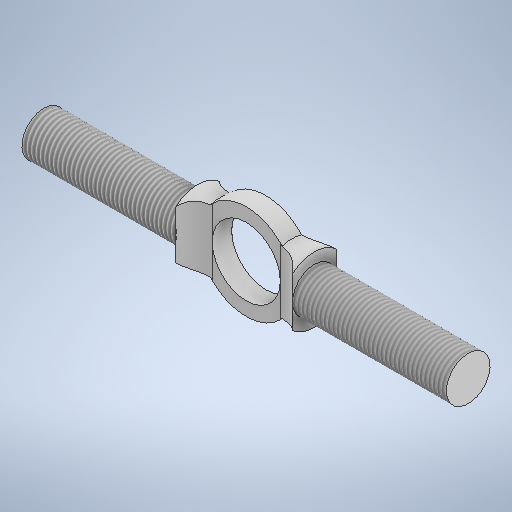
# Autodesk Inventor part: Schraubbolzen
Saved by Autodesk Inventor 2025.2 (Build 292293000, 293)
## iProperties
Created: 2025-02-03
Part Number: Schraubbolzen
Material: Generisch
Document SubType Name: Modeling
Designer: unter
Density: 1 g/cm^3
Appearance: Vorgabe
Author: unter
Autodesk Inventor part; units mm, degrees
ref_plane "YZ Plane" through (0, 0, 0) normal (1, 0, 0) x (0, 1, 0)
ref_plane "XZ Plane" through (0, 0, 0) normal (0, 1, 0) x (-1, 0, 0)
ref_plane "XY Plane" through (0, 0, 0) normal (0, 0, 1) x (1, 0, 0)
derived "Skelett_Laufkatze.ipt"
sketch "Schraubbolzen_oben" plane through (0, 0, -80) normal (0, 0, -1) x (-1, 0, 0)
  line L0 (181, -33.75) -> (131, -33.75) construction
  line L1 (131, -22.5) -> (181, -22.5) construction
  line L2 (131, 22.5) -> (181, 22.5) construction
  line L3 (131, 33.75) -> (181, 33.75) construction
  line L4 (-166, -33.75) -> (-116, -33.75) construction
  line L5 (-116, -22.5) -> (-166, -22.5) construction
  line L6 (-116, 22.5) -> (-166, 22.5) construction
  line L7 (-116, 33.75) -> (-166, 33.75) construction
  line L8 (218.5, 0) -> (-218.5, 0)
  circle A0 centre (0, 0) radius 35
  line L9 (218.5, 0) -> (218.5, 22.5)
  line L10 (218.5, 22.5) -> (60, 22.5)
  line L11 (60, 22.5) -> (60, 33.75)
  line L12 (60, 33.75) -> (36.8909, 33.75)
  line L13 (-36.8909, 33.75) -> (-60, 33.75)
  line L14 (-60, 33.75) -> (-60, 22.5)
  line L15 (-60, 22.5) -> (-218.5, 22.5)
  line L16 (-218.5, 22.5) -> (-218.5, 0)
  line L17 (0, 0) -> (0, 50) construction
  arc A1 (50, 0) -> (-50, 0) centre (0, 0) ccw
  point P0 (-35, 0)
  point P1 (35, 0)
sketch "Schraubbolzen_Ankerausschnitt" plane through (0, 0, -80) normal (0, 1, 0) x (-1, 0, 0)
  line L0 (218.5, 0) -> (-218.5, 0) construction
  line L1 (-35, 0) -> (35, 0) construction
  line L2 (60, 0) -> (36.8909, 0) construction
  line L3 (35, 10) -> (-35, 10)
  line L4 (-35, 10) -> (-35, -10)
  line L5 (-35, -10) -> (35, -10)
  line L6 (35, -10) -> (35, 10)
  line L7 (0, 10) -> (0, -10) construction
  arc A0 (35, 10) -> (60, 22.5) centre (35, 41.25) ccw
  arc A1 (60, -22.5) -> (35, -10) centre (35, -41.25) ccw
  arc A2 (-60, 22.5) -> (-35, 10) centre (-35, 41.25) ccw
  arc A3 (-35, -10) -> (-60, -22.5) centre (-35, -41.25) ccw
  line L8 (60, 22.5) -> (60, 41.25)
  line L9 (60, 41.25) -> (-60, 41.25)
  line L10 (-60, 41.25) -> (-60, 22.5)
  line L11 (60, -22.5) -> (60, -41.25)
  line L12 (60, -41.25) -> (-60, -41.25)
  line L13 (-60, -41.25) -> (-60, -22.5)
  point P0 (0, 80)
  point P1 (-60, 0)
  point P2 (0, 0)
revolve "Umdrehung1" add sketch "Schraubbolzen_oben" angle 360 about axis through (-218.5, 0, -80) along (1, 0, 0) contours L8 A1 L12 L11 L10 L9 | L8 A0 A1 | A1 L8 L16 L15 L14 L13
extrude "Extrusion1" cut sketch "Schraubbolzen_oben" along normal through all both and the other way through all contours A0 L8 | L8 A0
extrude "Extrusion2" cut sketch "Schraubbolzen_Ankerausschnitt" along normal through all both and the other way through all contours L3 A2 L10 L9 L8 A0 | A1 L11 L12 L13 A3 L5
thread "Gewinde1" size "M45x4.5" class "6g" standard "ANSI Metric M Profile" full length
thread "Gewinde2" size "M45x4.5" class "6g" standard "ANSI Metric M Profile" full length
